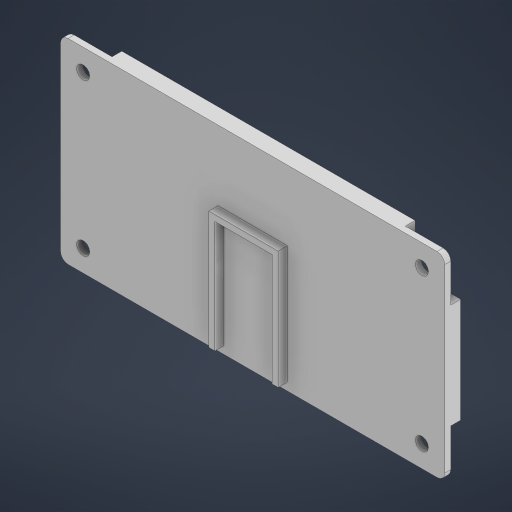
# Autodesk Inventor part: KeypadBase
Saved by Autodesk Inventor 2024.3 (Build 283343000, 343)
## iProperties
Created: 2025-12-23
Part Number: KeypadBase
Material: Generic
Document SubType Name: Modeling
Designer: zokur
Density: 1 g/cm^3
Appearance: Default
Author: zokur
Autodesk Inventor part; units mm, degrees
ref_plane "YZ Plane" through (0, 0, 0) normal (1, 0, 0) x (0, 1, 0)
ref_plane "XZ Plane" through (0, 0, 0) normal (0, 1, 0) x (-1, 0, 0)
ref_plane "XY Plane" through (0, 0, 0) normal (0, 0, 1) x (1, 0, 0)
sketch "Sketch1" plane through (0, 0, 0) normal (0, 0, 1) x (1, 0, 0)
  line L0 (0, 0) -> (126.85, 0)
  line L1 (126.85, 0) -> (126.85, 64.605)
  line L2 (126.85, 64.605) -> (0, 64.605)
  line L3 (0, 64.605) -> (0, 0)
  line L4 (55.925, 0) -> (65.5708, 0)
  line L5 (53.975, 0) -> (72.875, 0)
  line L6 (72.875, 0) -> (72.875, 39.5)
  line L7 (72.875, 39.5) -> (53.975, 39.5)
  line L8 (53.975, 39.5) -> (53.975, 0)
  line L9 (51.975, 0) -> (74.875, 0)
  line L10 (74.875, 0) -> (74.875, 41.5)
  line L11 (74.875, 41.5) -> (51.975, 41.5)
  line L12 (51.975, 41.5) -> (51.975, 0)
  point P0 (74.875, 20.75)
  point P1 (74.875, 0)
  dimension "d0" = 126.85
  dimension "d1" = 64.605
  dimension "d3" = 39.5
  dimension "d4" = 18.9
  dimension "d5" = 53.975
  dimension "d6" = 2
  dimension "d7" = 2
  dimension "d8" = 2
  constraints: 26 end point, 6 parallel, 4 horizontal, 3 perpendicular, 3 point on line, 1 midpoint
  measures "d0" distance of L1.end L2.end
  measures "d1" distance of L0.end L1.end
  measures "d3" distance of L5.end L6.end
  measures "d4" distance of L6.end L7.end
  measures "d5" distance between parallel lines of L3 L8
  measures "d6" distance between parallel lines of L7 L11
  measures "d7" distance from line of point (74.875, 20.75) L6
  measures "d8" distance between parallel lines of L8 L12
extrude "Extrusion2" add sketch "Sketch1" along normal blind 5.235 contours L3 L2 L1 L0 L10 L11 L12
extrude "Extrusion3" add sketch "Sketch1" along normal blind 8.235 contours L12 L11 L10 L0 L6 L7 L8
extrude "Extrusion4" add sketch "Sketch1" along normal blind 5.235 contours L8 L7 L6 L0
sketch "Sketch2" plane through (0, 0, 8.235) normal (0, 0, 1) x (1, 0, 0)
  line L0 (72.875, 39.5) -> (72.875, 0) projected
  line L1 (72.875, 0) -> (74.875, 0) projected
  line L2 (74.875, 0) -> (74.875, 41.5) projected
  line L3 (74.875, 41.5) -> (51.975, 41.5) projected
  line L4 (51.975, 41.5) -> (51.975, 0) projected
  line L5 (51.975, 0) -> (53.975, 0) projected
  line L6 (53.975, 0) -> (53.975, 39.5) projected
  line L7 (53.975, 39.5) -> (72.875, 39.5) projected
  line L8 (51.975, 0) -> (53.975, 0)
  line L9 (53.975, 0) -> (53.975, 2.5)
  line L10 (53.975, 2.5) -> (51.975, 2.5)
  line L11 (51.975, 2.5) -> (51.975, 0)
  line L12 (72.875, 0) -> (74.875, 0)
  line L13 (74.875, 0) -> (74.875, 2.5)
  line L14 (74.875, 2.5) -> (72.875, 2.5)
  line L15 (72.875, 2.5) -> (72.875, 0)
  point P0 (0, 0)
  dimension "d17" = 2.5
  dimension "d18" = 2.5
  constraints: 16 end point, 4 parallel, 2 horizontal, 2 perpendicular, 2 point on line
  measures "d17" distance between parallel lines of L5 L10
  measures "d18" distance between parallel lines of L1 L14
extrude "Extrusion5" cut sketch "Sketch2" against normal blind 3 contours L14 L2 L1 L0 | L6 L5 L4 L10
fillet "Fillet1" radius 2.5 4 edges at (126.85, 0, 2.6175) (0, 0, 2.6175) (126.85, 64.605, 2.6175) (0, 64.605, 2.6175)
sketch "Sketch3" plane through (0, 0, 5.235) normal (0, 0, 1) x (1, 0, 0)
  line L0 (0, 0) -> (15, 0)
  line L1 (15, 0) -> (15, 15)
  line L2 (15, 15) -> (0, 15)
  line L3 (0, 15) -> (0, 0)
  line L4 (0, 64.605) -> (15, 64.605)
  line L5 (15, 64.605) -> (15, 49.605)
  line L6 (15, 49.605) -> (0, 49.605)
  line L7 (0, 49.605) -> (0, 64.605)
  line L8 (124.35, 0) -> (2.5, 0) projected
  line L9 (126.85, 2.5) -> (126.85, 62.105) projected
  line L10 (126.85, 15) -> (111.85, 15)
  line L11 (111.85, 15) -> (111.85, 0)
  line L12 (111.85, 0) -> (126.85, 0)
  line L13 (126.85, 0) -> (126.85, 15)
  line L14 (126.85, 64.605) -> (111.85, 64.605)
  line L15 (111.85, 64.605) -> (111.85, 49.605)
  line L16 (111.85, 49.605) -> (126.85, 49.605)
  line L17 (126.85, 49.605) -> (126.85, 64.605)
  circle A0 centre (7.5, 57.44) radius 2.15
  circle A1 centre (119.35, 57.44) radius 2.15
  circle A2 centre (119.35, 7.165) radius 2.15
  line L18 (0, 62.105) -> (0, 2.5) projected
  circle A3 centre (7.5, 7.165) radius 2.15
  point P0 (111.85, 7.5)
  point P1 (119.35, 0)
  point P2 (119.35, 15)
  point P3 (7.5, 64.605)
  dimension "d22" = 15
  dimension "d23" = 15
  dimension "d24" = 15
  dimension "d25" = 15
  dimension "d26" = 64.605
  dimension "d28" = 15
  dimension "d29" = 15
  dimension "d30" = 15
  dimension "d31" = 15
  dimension "d32" = 64.605
  dimension "d33" = 0
  dimension "d52" = 7.165
  dimension "d53" = 7.5
  dimension "d54" = 4.3
  dimension "d55" = 4.3
  dimension "d56" = 7.5
  dimension "d57" = 7.165
  dimension "d58" = 4.3
  dimension "d59" = 7.5
  dimension "d61" = 7.165
  dimension "d62" = 0
  dimension "d63" = 4.3
  dimension "d65" = 7.5
  dimension "d66" = 7.165
  constraints: 32 end point, 8 parallel, 4 centre point, 4 horizontal, 4 midpoint, 4 perpendicular, 2 point on line
  measures "d22" distance of L0.end L1.end
  measures "d23" distance between parallel lines of L3 L1
  measures "d24" distance of L4.end L5.end
  measures "d25" distance between parallel lines of L7 L5
  measures "d26" distance between parallel lines of L8 L4
  measures "d28" distance from line of point (111.85, 7.5) L9
  measures "d29" distance of point (119.35, 0) point (119.35, 15)
  measures "d30" distance of L15.end L16.end
  measures "d31" distance of L16.end L14.start
  measures "d32" distance between parallel lines of L8 L14
  measures "d33" distance between parallel lines of L17 L9
  measures "d52" distance of A0.centre point (7.5, 64.605)
  measures "d53" distance from line of A0.centre L7
  measures "d54" diameter of A0
  measures "d55" diameter of A1
  measures "d56" distance from line of L17 A1.centre
  measures "d57" distance from line of L14 A1.centre
  measures "d58" diameter of A2
  measures "d59" distance from line of L9 A2.centre
  measures "d61" distance from line of A2.centre L8
  measures "d62" distance between parallel lines of L18 L7
  measures "d63" diameter of A3
  measures "d65" distance from line of A3.centre L18
  measures "d66" distance from line of L8 A3.centre
sketch "Sketch4" plane through (0, 0, 0) normal (0, 0, -1) x (-1, 0, 0)
  line L0 (-126.85, 0) -> (-111.85, 0)
  line L1 (-111.85, 0) -> (-111.85, 15)
  line L2 (-111.85, 15) -> (-126.85, 15)
  line L3 (-126.85, 15) -> (-126.85, 0)
  line L4 (-126.85, 64.605) -> (-111.85, 64.605)
  line L5 (-111.85, 64.605) -> (-111.85, 49.605)
  line L6 (-111.85, 49.605) -> (-126.85, 49.605)
  line L7 (-126.85, 49.605) -> (-126.85, 64.605)
  line L8 (-85.2582, 0) -> (-207.1082, 0)
  line L9 (0, -43.3004) -> (0, 16.3046)
  line L10 (0, 15) -> (-15, 15)
  line L11 (-15, 15) -> (-15, 0)
  line L12 (-15, 0) -> (0, 0)
  line L13 (0, 0) -> (0, 15)
  line L14 (0, 64.605) -> (-15, 64.605)
  line L15 (-15, 64.605) -> (-15, 49.605)
  line L16 (-15, 49.605) -> (0, 49.605)
  line L17 (0, 49.605) -> (0, 64.605)
  line L18 (-2.5, 0) -> (-124.35, 0) projected
  line L19 (0, 62.105) -> (0, 2.5) projected
  line L20 (-126.85, 2.5) -> (-126.85, 62.105) projected
  point P0 (0, 0)
  point P1 (-15, 7.5)
  point P2 (-7.5, 0)
  point P3 (-7.5, 15)
  point P4 (0, 32.3025)
  point P5 (-119.35, 0)
  dimension "d34" = 15
  dimension "d35" = 15
  dimension "d36" = 15
  dimension "d37" = 15
  dimension "d38" = 64.605
  dimension "d39" = 0
  dimension "d40" = 15
  dimension "d41" = 15
  dimension "d42" = 15
  dimension "d43" = 15
  dimension "d44" = 64.605
  dimension "d45" = 0
  dimension "d46" = 0
  dimension "d47" = 0
  dimension "d48" = 0
  dimension "d49" = 0
  constraints: 36 end point, 8 parallel, 5 midpoint, 4 horizontal, 4 perpendicular, 2 point on line
  measures "d34" distance of L1.start L1.end
  measures "d35" distance between parallel lines of L3 L1
  measures "d36" distance of L5.start L5.end
  measures "d37" distance between parallel lines of L7 L5
  measures "d38" distance between parallel lines of L8 L4
  measures "d39" distance between parallel lines of L5 L1
  measures "d40" distance from line of point (-15, 7.5) L9
  measures "d41" distance of point (-7.5, 0) point (-7.5, 15)
  measures "d42" distance of L15.end L17.start
  measures "d43" distance of L17.start L14.start
  measures "d44" distance between parallel lines of L8 L14
  measures "d45" distance between parallel lines of L17 L9
  measures "d46" distance between parallel lines of L18 L8
  measures "d47" distance from line of point (0, 32.303) L9
  measures "d48" distance between parallel lines of L20 L3
  measures "d49" distance from line of L18 point (-119.35, 0)
extrude "Extrusion6" cut sketch "Sketch4" against normal blind 3.235
extrude "Extrusion7" cut sketch "Sketch3" against normal blind 3.235 contours A0 | A1 | A2 | A3
body "Solid2"
